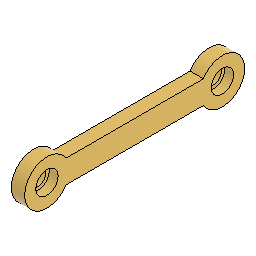
06 Link (Autodesk Fusion 360 design; units mm, degrees)
Autodesk Fusion 360 part; units mm, degrees
note: some values were not read from the file. Set by a fixed rule: which sketch regions a step uses.
sketch "Boceto1" plane through (0, 0, 0) normal (1, 0, 0) x (0, 1, 0)
  line L0 (107.0846, 27.5) -> (140.003, 49.1343) construction
  line L1 (112.0816, 27.6728) -> (137.8619, 44.6159)
  line L2 (109.2257, 32.0184) -> (135.0059, 48.9614)
  circle A0 centre (140.003, 49.1343) radius 1.75
  arc A1 (137.8619, 44.6159) -> (135.0059, 48.9614) centre (140.003, 49.1343) ccw
  arc A2 (109.2257, 32.0184) -> (112.0816, 27.6728) centre (107.0846, 27.5) ccw
  circle A3 centre (107.0846, 27.5) radius 1.75
  dimension "d199" = 10
  dimension "d204" = 3.5
  dimension "d205" = 10
  dimension "d206" = 3.5
  constraint coincident L0.start A2.centre
  constraint coincident L0.end A0.centre
  constraint concentric A0 A1
  constraint concentric A2 A3
  measures "d199" diameter of A2
  measures "d204" diameter of A0
  measures "d205" diameter of A1
  measures "d206" diameter of A3
extrude "Extruir1" add sketch "Boceto1" along normal blind 3
move_body "Desplazar1" bodies 1 to x (1, 0, 0) y (0, 1, 0) z (0, 0, 1) at (-3, -107.0846, -27.5)
move_body "Desplazar2" bodies 1 to x (1, 0, 0) y (0, 0.835807, -0.549023) z (0, 0.549023, 0.835807) at (0, 0, 0)
hole "Agujero1" at (0, 0, 0) direction (-1, 0, 0) diameter 3 depth 14 tip angle 180 counterbore diameter 5 counterbore depth 2
hole "Agujero2" at (0, 39.3911, 0.0091) direction (-1, 0, 0) diameter 3 depth 14 tip angle 180 counterbore diameter 5 counterbore depth 2
mirror "Simetría1" [suppressed]
named bodies: "Link"
